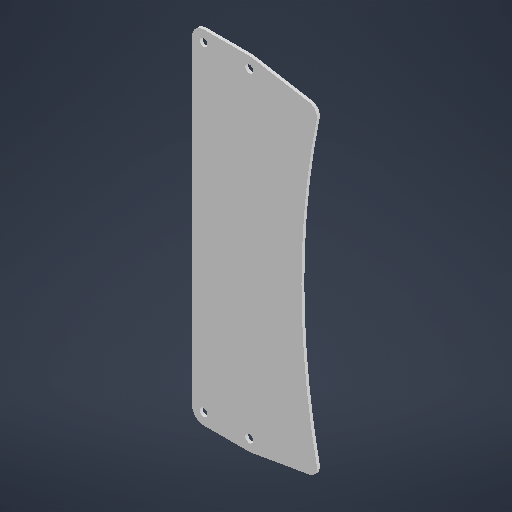
# Autodesk Inventor part: wedge
Saved by Autodesk Inventor 2025.1 (Build 291241000, 241)
## iProperties
Created: 2025-01-15
Part Number: wedge
Material: Generic
Document SubType Name: Modeling
Designer: Jahan
Density: 1 g/cm^3
Appearance: Default
Author: Jahan
Autodesk Inventor part; units mm, degrees
ref_plane "YZ Plane" through (0, 0, 0) normal (1, 0, 0) x (0, 1, 0)
ref_plane "XZ Plane" through (0, 0, 0) normal (0, 1, 0) x (-1, 0, 0)
ref_plane "XY Plane" through (0, 0, 0) normal (0, 0, 1) x (1, 0, 0)
sketch "Sketch1" plane through (0, 0, 0) normal (0, 0, 1) x (1, 0, 0)
  circle A0 centre (-39.5621, -80.6318) radius 2.1844
  circle A1 centre (-14.1621, -80.6318) radius 2.1844
  circle A2 centre (-14.1621, 97.1682) radius 2.1844
  circle A3 centre (-39.5621, 97.1682) radius 2.1844
  arc A4 (19.2671, -81.2453) -> (23.3688, -75.2127) centre (18.394, -76.2409) ccw
  line L0 (19.2671, -81.2453) -> (-13.0707, -86.8873)
  arc A5 (14.8318, 8.2682) -> (23.3688, -75.2127) centre (427.2689, 8.2682) ccw
  arc A6 (23.3688, 91.749) -> (14.8318, 8.2682) centre (427.2689, 8.2682) ccw
  arc A7 (23.3688, 91.749) -> (19.2671, 97.7816) centre (18.394, 92.7772) ccw
  line L1 (19.2671, 97.7816) -> (-13.0707, 103.4237)
  line L2 (-39.5621, -86.9818) -> (-14.1621, -86.9818)
  line L3 (-14.1621, 103.5182) -> (-39.5621, 103.5182)
  line L4 (-45.9121, -80.6318) -> (-45.9121, 97.1682)
  arc A8 (-45.9121, -80.6318) -> (-39.5621, -86.9818) centre (-39.5621, -80.6318) ccw
  arc A9 (-14.1621, -86.9818) -> (-13.0707, -86.8873) centre (-14.1621, -80.6318) ccw
  arc A10 (-13.0707, 103.4237) -> (-14.1621, 103.5182) centre (-14.1621, 97.1682) ccw
  arc A11 (-39.5621, 103.5182) -> (-45.9121, 97.1682) centre (-39.5621, 97.1682) ccw
  point P0 (0, 0)
  dimension "d0" = 5.08
  constraints: 16 point on circle, 12 centre point, 10 end point, 4 coincident, 1 horizontal, 1 tangent
  measures "d0" radius of A4
extrude "Extrusion1" add sketch "Sketch1" along normal blind 1.5875
body "Solid1"
